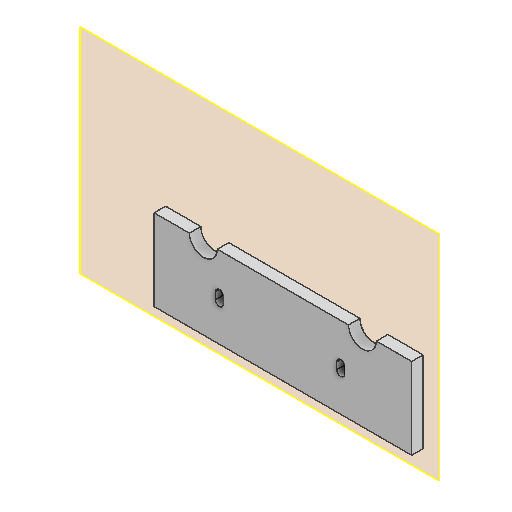
# Autodesk Inventor part: Part5
Saved by Autodesk Inventor 2025.1 (Build 291241020, 241B)
## iProperties
Created: 2024-09-24
Part Number: Part5
Material: Generic
Document SubType Name: Modeling
Designer: wayneslade
Density: 1 g/cm^3
Appearance: Default
Author: wayneslade
Autodesk Inventor part; units mm, degrees
ref_plane "YZ Plane" through (0, 0, 0) normal (1, 0, 0) x (0, 1, 0)
ref_plane "XZ Plane" through (0, 0, 0) normal (0, 1, 0) x (-1, 0, 0)
ref_plane "XY Plane" through (0, 0, 0) normal (0, 0, 1) x (1, 0, 0)
ref_plane "Work Plane1" through (0, 0, 0) normal (0, 0, 1) x (1, 0, 0)
sketch "Sketch1" plane through (0, 0, 0) normal (0, 0, 1) x (1, 0, 0)
  line L0 (22.8064, -35.5) -> (-89.6938, -35.5)
  line L1 (-89.6938, -35.5) -> (-89.6938, 0)
  line L2 (-89.6938, 0) -> (-74.2938, 0)
  line L3 (22.8064, 0) -> (22.8064, -35.5)
  circle A0 centre (11.5562, -18) radius 2 construction
  line L4 (-53.1938, -16) -> (-53.1938, -30) construction
  arc A1 (-56.1938, -30) -> (-53.1938, -30) centre (-54.6938, -30) ccw construction
  line L5 (-56.1938, -30) -> (-56.1938, -16) construction
  arc A2 (-53.1938, -16) -> (-56.1938, -16) centre (-54.6938, -16) ccw construction
  line L6 (7.0562, -16) -> (7.0562, -30) construction
  arc A3 (4.0562, -30) -> (7.0562, -30) centre (5.5562, -30) ccw construction
  line L7 (4.0562, -30) -> (4.0562, -16) construction
  arc A4 (7.0562, -16) -> (4.0562, -16) centre (5.5562, -16) ccw construction
  line L8 (-13.1938, -16) -> (-13.1938, -30) construction
  arc A5 (-16.1938, -30) -> (-13.1938, -30) centre (-14.6938, -30) ccw construction
  line L9 (-16.1938, -30) -> (-16.1938, -16) construction
  arc A6 (-13.1938, -16) -> (-16.1938, -16) centre (-14.6938, -16) ccw construction
  arc A7 (19.0562, -16) -> (16.0562, -16) centre (17.5562, -16) ccw construction
  line L10 (19.0562, -16) -> (19.0562, -30) construction
  arc A8 (16.0562, -30) -> (19.0562, -30) centre (17.5562, -30) ccw construction
  line L11 (16.0562, -30) -> (16.0562, -16) construction
  line L12 (22.8064, -40) -> (22.8064, 45) construction
  line L13 (22.8064, 45) -> (-120, 45) construction
  line L14 (-120, 27.5563) -> (-120, 45) construction
  line L15 (-120, 27.5563) -> (-95.2035, 27.5563) construction
  arc A9 (-85.0841, 27.5563) -> (-95.2035, 27.5563) centre (-90.1438, 25.4) ccw construction
  line L16 (-85.0841, 27.5563) -> (17.8062, 27.5563) construction
  line L17 (17.8062, 27.5563) -> (17.8062, -11) construction
  line L18 (17.8062, -11) -> (-120, -11) construction
  line L19 (-120, -40) -> (-120, -11) construction
  line L20 (22.8064, -40) -> (-120, -40) construction
  circle A10 centre (-111.1938, -18) radius 2 construction
  circle A11 centre (-98.1938, -18) radius 2 construction
  circle A12 centre (-61.1938, -18) radius 2 construction
  circle A13 centre (-48.1938, -18) radius 2 construction
  circle A14 centre (-21.1938, -18) radius 2 construction
  circle A15 centre (-8.1938, -18) radius 2 construction
  circle A16 centre (-21.1938, 33.6563) radius 2 construction
  circle A17 centre (-8.1938, 33.6563) radius 2 construction
  circle A18 centre (-61.1938, 33.6563) radius 2 construction
  circle A19 centre (-48.1938, 33.6563) radius 2 construction
  circle A20 centre (-111.1938, 33.6563) radius 2 construction
  circle A21 centre (-98.1938, 33.6563) radius 2 construction
  circle A22 centre (-90.1438, -25.4) radius 5.5 construction
  line L21 (-84.6938, 26.6563) -> (-89.6938, 26.6563) construction
  line L22 (-89.6938, 26.6563) -> (-89.6938, -11) construction
  line L23 (-84.6938, -11) -> (-89.6938, -11) construction
  line L24 (-84.6938, 26.6563) -> (-84.6938, -11) construction
  line L25 (-84.6938, 26.6563) -> (-84.6938, -11) construction
  circle A23 centre (1.3062, 0) radius 6 construction
  circle A24 centre (-68.1938, 0) radius 6 construction
  arc A25 (-4.7938, 0) -> (7.4062, 0) centre (1.3062, 0) ccw
  arc A26 (-74.2938, 0) -> (-62.0938, 0) centre (-68.1938, 0) ccw
  line L26 (-148.5613, 0) -> (51.3677, 0) construction
  line L27 (7.4062, 0) -> (22.8064, 0)
  line L28 (-62.0938, 0) -> (-4.7938, 0)
  point P0 (0, 0)
  point P1 (17.5562, -31.5)
  dimension "d0" = 0
  dimension "d1" = 0
  dimension "d2" = 4
  dimension "d3" = 0.1
  dimension "d4" = 0.1
  constraints: 12 end point, 5 point on circle, 4 parallel, 3 collinear, 2 centre point, 2 coincident, 2 point on line, 1 horizontal, 1 perpendicular
  measures "d0" distance between parallel lines of L22 L1
  measures "d1" distance between parallel lines of L12 L3
  measures "d2" distance from line of L0 point (17.556, -31.5)
  measures "d3" radial gap between concentric circles of A23 A25
  measures "d4" radial gap between concentric circles of A24 A26
extrude "Main Body" add sketch "Sketch1" along normal blind 5
sketch "Sketch2" plane through (0, 0, 0) normal (0, 0, -1) x (-1, 0, 0)
  line L0 (56.1938, -30) -> (56.1938, -16) construction
  arc A0 (53.1938, -30) -> (56.1938, -30) centre (54.6938, -30) ccw construction
  line L1 (53.1938, -16) -> (53.1938, -30) construction
  arc A1 (56.1938, -16) -> (53.1938, -16) centre (54.6938, -16) ccw construction
  arc A2 (13.1938, -30) -> (16.1938, -30) centre (14.6938, -30) ccw construction
  line L2 (13.1938, -16) -> (13.1938, -30) construction
  arc A3 (16.1938, -16) -> (13.1938, -16) centre (14.6938, -16) ccw construction
  line L3 (16.1938, -30) -> (16.1938, -16) construction
  line L4 (14.6938, -16) -> (14.6938, -30) construction
  line L5 (54.6938, -16) -> (54.6938, -30) construction
  line L6 (14.6938, -29) -> (14.6938, -17) construction
  line L7 (13.2438, -29) -> (13.2438, -17)
  line L8 (16.1438, -17) -> (16.1438, -29)
  arc A4 (13.2438, -29) -> (16.1438, -29) centre (14.6938, -29) ccw
  arc A5 (16.1438, -17) -> (13.2438, -17) centre (14.6938, -17) ccw
  line L9 (54.6938, -29) -> (54.6938, -17) construction
  line L10 (53.2438, -29) -> (53.2438, -17)
  line L11 (56.1438, -17) -> (56.1438, -29)
  arc A6 (53.2438, -29) -> (56.1438, -29) centre (54.6938, -29) ccw
  arc A7 (56.1438, -17) -> (53.2438, -17) centre (54.6938, -17) ccw
  line L12 (14.6938, -17) -> (54.6938, -17) construction
  point P0 (0, 0)
  point P1 (14.6938, -23)
  point P2 (54.6938, -23)
  dimension "d7" = 0.05
  dimension "d8" = 0.05
  dimension "d9" = 1
  constraints: 22 end point, 8 point on circle, 8 tangent, 4 centre point, 4 midpoint, 2 parallel, 2 point on line, 2 vertical, 1 horizontal
  measures "d7" distance between parallel lines of L3 L8
  measures "d8" distance between parallel lines of L1 L10
  measures "d9" distance of L4.start L6.end
extrude "Alignment Tabs" add sketch "Sketch2" along normal blind 1.8
sketch "Sketch3" plane through (0, 0, 5) normal (0, 0, -1) x (-1, 0, 0)
  circle A0 centre (61.1938, -18) radius 2 construction
  circle A1 centre (8.1938, -18) radius 2 construction
  line L0 (61.1938, -16.5) -> (61.1938, -19.5) construction
  line L1 (59.4438, -16.5) -> (59.4438, -19.5)
  line L2 (62.9438, -19.5) -> (62.9438, -16.5)
  arc A2 (62.9438, -16.5) -> (59.4438, -16.5) centre (61.1938, -16.5) ccw
  arc A3 (59.4438, -19.5) -> (62.9438, -19.5) centre (61.1938, -19.5) ccw
  line L3 (8.1938, -16.5) -> (8.1938, -19.5) construction
  line L4 (6.4438, -16.5) -> (6.4438, -19.5)
  line L5 (9.9438, -19.5) -> (9.9438, -16.5)
  arc A4 (9.9438, -16.5) -> (6.4438, -16.5) centre (8.1938, -16.5) ccw
  arc A5 (6.4438, -19.5) -> (9.9438, -19.5) centre (8.1938, -19.5) ccw
  point P0 (0, 0)
  dimension "d12" = 3.5
  dimension "d13" = 3.5
  dimension "d14" = 3
  dimension "d15" = 3
  constraints: 16 end point, 8 point on circle, 8 tangent, 4 centre point, 3 parallel, 2 midpoint, 1 vertical
  measures "d12" distance between parallel lines of L1 L2
  measures "d13" distance between parallel lines of L4 L5
  measures "d14" distance of L0.end L0.start
  measures "d15" distance of L3.end L3.start
extrude "Slots for Screws M3" cut sketch "Sketch3" along normal through all
equation "\"d4\" = d3"
equation "\"d8\" = d7"
equation "\"d13\" = d12"
equation "\"d15\" = d14"
body "Solid1"
